Autodesk Fusion 360 part; units mm, degrees
note: some values were not read from the file. Chosen so that the rebuilt part matches the saved one: which bodies a step acts on. Set by a fixed rule: which sketch regions a step uses.
(part 3 of 6)
sketch "Sketch73" plane through (0, 0, 40) normal (0, 0, 1) x (-1, 0, 0)
  line L0 (-70.6667, -90.7407) -> (-70.6667, -70.6667)
  line L1 (-70.6667, -70.6667) -> (-90.7407, -70.6667)
  line L2 (-90.7407, -70.6667) -> (-90.7407, -67.1667)
  line L3 (-90.7407, -67.1667) -> (-109.2593, -67.1667)
  line L4 (-109.2593, -67.1667) -> (-109.2593, -70.6667)
  line L5 (-109.2593, -70.6667) -> (-129.3333, -70.6667)
  line L6 (-129.3333, -70.6667) -> (-129.3333, -88.8889)
  line L7 (-129.3333, -88.8889) -> (-137.3333, -88.8889)
  line L8 (-137.3333, -88.8889) -> (-137.3333, -70.6667)
  line L9 (-137.3333, -70.6667) -> (-157.4074, -70.6667)
  line L10 (-157.4074, -70.6667) -> (-157.4074, -67.1667)
  line L11 (-157.4074, -67.1667) -> (-175.9259, -67.1667)
  line L12 (-175.9259, -67.1667) -> (-175.9259, -70.6667)
  line L13 (-175.9259, -70.6667) -> (-196, -70.6667)
  line L14 (-196, -70.6667) -> (-196, -88.8889)
  line L15 (-196, -88.8889) -> (-200, -88.8889)
  line L16 (-200, -88.8889) -> (-200, -111.1111)
  line L17 (-200, -111.1111) -> (-196, -111.1111)
  line L18 (-196, -111.1111) -> (-196, -129.3333)
  line L19 (-196, -129.3333) -> (-177.7778, -129.3333)
  line L20 (-177.7778, -129.3333) -> (-177.7778, -137.3333)
  line L21 (-177.7778, -137.3333) -> (-196, -137.3333)
  line L22 (-196, -137.3333) -> (-196, -155.5556)
  line L23 (-196, -155.5556) -> (-200, -155.5556)
  line L24 (-200, -155.5556) -> (-200, -177.7778)
  line L25 (-200, -177.7778) -> (-196, -177.7778)
  line L26 (-196, -177.7778) -> (-196, -196)
  line L27 (-196, -196) -> (-177.7778, -196)
  line L28 (-177.7778, -196) -> (-177.7778, -200)
  line L29 (-177.7778, -200) -> (-155.5556, -200)
  line L30 (-155.5556, -200) -> (-155.5556, -196)
  line L31 (-155.5556, -196) -> (-137.3333, -196)
  line L32 (-137.3333, -196) -> (-137.3333, -177.7778)
  line L33 (-137.3333, -177.7778) -> (-129.3333, -177.7778)
  line L34 (-129.3333, -177.7778) -> (-129.3333, -196)
  line L35 (-129.3333, -196) -> (-111.1111, -196)
  line L36 (-111.1111, -196) -> (-111.1111, -200)
  line L37 (-111.1111, -200) -> (-88.8889, -200)
  line L38 (-88.8889, -200) -> (-88.8889, -196)
  line L39 (-88.8889, -196) -> (-70.6667, -196)
  line L40 (-70.6667, -196) -> (-70.6667, -177.7778)
  line L41 (-70.6667, -177.7778) -> (-62.6667, -177.7778)
  line L42 (-62.6667, -177.7778) -> (-62.6667, -196)
  line L43 (-62.6667, -196) -> (-44.4444, -196)
  line L44 (-44.4444, -196) -> (-44.4444, -200)
  line L45 (-44.4444, -200) -> (-22.2222, -200)
  line L46 (-22.2222, -200) -> (-22.2222, -196)
  line L47 (-22.2222, -196) -> (-4, -196)
  line L48 (-4, -196) -> (-4, -177.7778)
  line L49 (-4, -177.7778) -> (0, -177.7778)
  line L50 (0, -177.7778) -> (0, -155.5556)
  line L51 (0, -155.5556) -> (-4, -155.5556)
  line L52 (-4, -155.5556) -> (-4, -137.3333)
  line L53 (-4, -137.3333) -> (-24.0741, -137.3333)
  line L54 (-24.0741, -137.3333) -> (-24.0741, -133.8333)
  line L55 (-24.0741, -133.8333) -> (-42.5926, -133.8333)
  line L56 (-42.5926, -133.8333) -> (-42.5926, -137.3333)
  line L57 (-42.5926, -137.3333) -> (-62.6667, -137.3333)
  line L58 (-62.6667, -137.3333) -> (-62.6667, -155.5556)
  line L59 (-62.6667, -155.5556) -> (-70.6667, -155.5556)
  line L60 (-70.6667, -155.5556) -> (-70.6667, -137.3333)
  line L61 (-70.6667, -137.3333) -> (-88.8889, -137.3333)
  line L62 (-88.8889, -137.3333) -> (-88.8889, -129.3333)
  line L63 (-88.8889, -129.3333) -> (-70.6667, -129.3333)
  line L64 (-70.6667, -129.3333) -> (-70.6667, -109.2593)
  line L65 (-70.6667, -109.2593) -> (-67.1667, -109.2593)
  line L66 (-67.1667, -109.2593) -> (-67.1667, -90.7407)
  line L67 (-67.1667, -90.7407) -> (-70.6667, -90.7407)
  line L68 (-129.3333, -137.3333) -> (-129.3333, -155.5556)
  line L69 (-129.3333, -155.5556) -> (-137.3333, -155.5556)
  line L70 (-137.3333, -155.5556) -> (-137.3333, -137.3333)
  line L71 (-137.3333, -137.3333) -> (-155.5556, -137.3333)
  line L72 (-155.5556, -137.3333) -> (-155.5556, -129.3333)
  line L73 (-155.5556, -129.3333) -> (-137.3333, -129.3333)
  line L74 (-137.3333, -129.3333) -> (-137.3333, -111.1111)
  line L75 (-137.3333, -111.1111) -> (-129.3333, -111.1111)
  line L76 (-129.3333, -111.1111) -> (-129.3333, -129.3333)
  line L77 (-129.3333, -129.3333) -> (-111.1111, -129.3333)
  line L78 (-111.1111, -129.3333) -> (-111.1111, -137.3333)
  line L79 (-111.1111, -137.3333) -> (-129.3333, -137.3333)
  line L80 (-88.8889, -137.3333) -> (-90.7407, -137.3333)
  line L81 (-90.7407, -137.3333) -> (-90.7407, -129.3333)
  line L82 (-90.7407, -129.3333) -> (-88.8889, -129.3333)
  line L83 (-88.8889, -129.3333) -> (-88.8889, -137.3333)
  line L84 (-111.1111, -137.3333) -> (-109.2593, -137.3333)
  line L85 (-109.2593, -137.3333) -> (-109.2593, -129.3333)
  line L86 (-109.2593, -129.3333) -> (-111.1111, -129.3333)
  line L87 (-111.1111, -129.3333) -> (-111.1111, -137.3333)
  line L88 (-88.8889, -133.8333) -> (-111.1111, -133.8333)
  line L89 (-111.1111, -133.8333) -> (-111.1111, -132.8333)
  line L90 (-111.1111, -132.8333) -> (-88.8889, -132.8333)
  line L91 (-88.8889, -132.8333) -> (-88.8889, -133.8333)
  line L92 (-129.3333, -111.1111) -> (-137.3333, -111.1111)
  line L93 (-137.3333, -111.1111) -> (-137.3333, -109.2593)
  line L94 (-137.3333, -109.2593) -> (-129.3333, -109.2593)
  line L95 (-129.3333, -109.2593) -> (-129.3333, -111.1111)
  line L96 (-129.3333, -88.8889) -> (-137.3333, -88.8889)
  line L97 (-137.3333, -88.8889) -> (-137.3333, -90.7407)
  line L98 (-137.3333, -90.7407) -> (-129.3333, -90.7407)
  line L99 (-129.3333, -90.7407) -> (-129.3333, -88.8889)
  line L100 (-132.8333, -111.1111) -> (-133.8333, -111.1111)
  line L101 (-133.8333, -111.1111) -> (-133.8333, -88.8889)
  line L102 (-133.8333, -88.8889) -> (-132.8333, -88.8889)
  line L103 (-132.8333, -88.8889) -> (-132.8333, -111.1111)
  dimension "d406" = 1.8519
  dimension "d407" = 1.8519
  dimension "d408" = 8
  dimension "d409" = 8
  dimension "d410" = 22.2222
  dimension "d411" = 1
  dimension "d412" = 3.5
  dimension "d413" = 8
  dimension "d414" = 1.8519
  dimension "d415" = 1.8519
  dimension "d416" = 8
  dimension "d421" = 1
  dimension "d422" = 3.5
  dimension "d423" = 22.2222
  constraint horizontal L80
  constraint vertical L81
  constraint horizontal L82
  constraint vertical L83
  constraint coincident L61.end L62.start
  constraint horizontal L84
  constraint vertical L85
  constraint horizontal L86
  constraint vertical L87
  constraint coincident L78.end L79.start
  constraint horizontal L88
  constraint vertical L89
  constraint horizontal L90
  constraint vertical L91
  constraint coincident L83 L88.start
  constraint horizontal L92
  constraint vertical L93
  constraint horizontal L94
  constraint vertical L95
  constraint coincident L75.end L76.start
  constraint horizontal L96
  constraint vertical L97
  constraint horizontal L98
  constraint vertical L99
  constraint coincident L6.end L7.start
  constraint horizontal L100
  constraint vertical L101
  constraint horizontal L102
  constraint vertical L103
  constraint coincident L75 L100.start
  measures "d406" distance of L81.end L62.end
  measures "d407" distance of L85.end L77.end
  measures "d408" distance of L78.end L77.end
  measures "d409" distance of L61.end L62.end
  measures "d410" distance of L89.end L90.end
  measures "d411" distance of L88.end L89.end
  measures "d412" distance of L78.end L88.end
  measures "d413" distance of L6.end L7.end
  measures "d414" distance of L7.end L97.end
  measures "d415" distance of L74.end L93.end
  measures "d416" distance of L93.end L94.end
  measures "d421" distance of L101.end L102.end
  measures "d422" distance of L6.end L103
  measures "d423" distance of L100.end L101.end
extrude "Extrude42" cut sketch "Sketch73" against normal blind 4 contours L62 L81 L82 L83 L90 | L62 L81 L83 L88 L90 L91 | L7 L96 L98 L99 L103 | L62 L80 L81 L83 L88 | L81 L85 L88 L90 | L7 L96 L98 L101 L102 L103 | L78 L85 L86 L87 L90 | L78 L85 L87 L88 L89 L90 | L7 L96 L97 L98 L101 | L94 L98 L101 L103 | L78 L84 L85 L87 L88 | L75 L92 L94 L100 L101 L103 | L75 L92 L94 L95 L103 | L75 L92 L93 L94 L101 bodies 17 makes body 18 at (163.679, 103.0864, 40)
sketch "Sketch74" plane through (0, 0, 40) normal (0, 0, 1) x (-1, 0, 0)
  line L0 (-109.2593, -137.3333) -> (-129.3333, -137.3333)
  line L1 (-129.3333, -137.3333) -> (-129.3333, -155.5556)
  line L2 (-129.3333, -155.5556) -> (-137.3333, -155.5556)
  line L3 (-137.3333, -155.5556) -> (-137.3333, -137.3333)
  line L4 (-137.3333, -137.3333) -> (-155.5556, -137.3333)
  line L5 (-155.5556, -137.3333) -> (-155.5556, -129.3333)
  line L6 (-155.5556, -129.3333) -> (-137.3333, -129.3333)
  line L7 (-137.3333, -129.3333) -> (-137.3333, -109.2593)
  line L8 (-137.3333, -109.2593) -> (-133.8333, -109.2593)
  line L9 (-133.8333, -109.2593) -> (-133.8333, -90.7407)
  line L10 (-133.8333, -90.7407) -> (-137.3333, -90.7407)
  line L11 (-137.3333, -90.7407) -> (-137.3333, -70.6667)
  line L12 (-137.3333, -70.6667) -> (-157.4074, -70.6667)
  line L13 (-157.4074, -70.6667) -> (-157.4074, -67.1667)
  line L14 (-157.4074, -67.1667) -> (-175.9259, -67.1667)
  line L15 (-175.9259, -67.1667) -> (-175.9259, -70.6667)
  line L16 (-175.9259, -70.6667) -> (-196, -70.6667)
  line L17 (-196, -70.6667) -> (-196, -88.8889)
  line L18 (-196, -88.8889) -> (-200, -88.8889)
  line L19 (-200, -88.8889) -> (-200, -111.1111)
  line L20 (-200, -111.1111) -> (-196, -111.1111)
  line L21 (-196, -111.1111) -> (-196, -129.3333)
  line L22 (-196, -129.3333) -> (-177.7778, -129.3333)
  line L23 (-177.7778, -129.3333) -> (-177.7778, -137.3333)
  line L24 (-177.7778, -137.3333) -> (-196, -137.3333)
  line L25 (-196, -137.3333) -> (-196, -155.5556)
  line L26 (-196, -155.5556) -> (-200, -155.5556)
  line L27 (-200, -155.5556) -> (-200, -177.7778)
  line L28 (-200, -177.7778) -> (-196, -177.7778)
  line L29 (-196, -177.7778) -> (-196, -196)
  line L30 (-196, -196) -> (-177.7778, -196)
  line L31 (-177.7778, -196) -> (-177.7778, -200)
  line L32 (-177.7778, -200) -> (-155.5556, -200)
  line L33 (-155.5556, -200) -> (-155.5556, -196)
  line L34 (-155.5556, -196) -> (-137.3333, -196)
  line L35 (-137.3333, -196) -> (-137.3333, -177.7778)
  line L36 (-137.3333, -177.7778) -> (-129.3333, -177.7778)
  line L37 (-129.3333, -177.7778) -> (-129.3333, -196)
  line L38 (-129.3333, -196) -> (-111.1111, -196)
  line L39 (-111.1111, -196) -> (-111.1111, -200)
  line L40 (-111.1111, -200) -> (-88.8889, -200)
  line L41 (-88.8889, -200) -> (-88.8889, -196)
  line L42 (-88.8889, -196) -> (-70.6667, -196)
  line L43 (-70.6667, -196) -> (-70.6667, -177.7778)
  line L44 (-70.6667, -177.7778) -> (-62.6667, -177.7778)
  line L45 (-62.6667, -177.7778) -> (-62.6667, -196)
  line L46 (-62.6667, -196) -> (-44.4444, -196)
  line L47 (-44.4444, -196) -> (-44.4444, -200)
  line L48 (-44.4444, -200) -> (-22.2222, -200)
  line L49 (-22.2222, -200) -> (-22.2222, -196)
  line L50 (-22.2222, -196) -> (-4, -196)
  line L51 (-4, -196) -> (-4, -177.7778)
  line L52 (-4, -177.7778) -> (0, -177.7778)
  line L53 (0, -177.7778) -> (0, -155.5556)
  line L54 (0, -155.5556) -> (-4, -155.5556)
  line L55 (-4, -155.5556) -> (-4, -137.3333)
  line L56 (-4, -137.3333) -> (-24.0741, -137.3333)
  line L57 (-24.0741, -137.3333) -> (-24.0741, -133.8333)
  line L58 (-24.0741, -133.8333) -> (-42.5926, -133.8333)
  line L59 (-42.5926, -133.8333) -> (-42.5926, -137.3333)
  line L60 (-42.5926, -137.3333) -> (-62.6667, -137.3333)
  line L61 (-62.6667, -137.3333) -> (-62.6667, -155.5556)
  line L62 (-62.6667, -155.5556) -> (-70.6667, -155.5556)
  line L63 (-70.6667, -155.5556) -> (-70.6667, -137.3333)
  line L64 (-70.6667, -137.3333) -> (-90.7407, -137.3333)
  line L65 (-90.7407, -137.3333) -> (-90.7407, -133.8333)
  line L66 (-90.7407, -133.8333) -> (-109.2593, -133.8333)
  line L67 (-109.2593, -133.8333) -> (-109.2593, -137.3333)
  line L68 (-155.5556, -137.3333) -> (-157.4074, -137.3333)
  line L69 (-157.4074, -137.3333) -> (-157.4074, -129.3333)
  line L70 (-157.4074, -129.3333) -> (-155.5556, -129.3333)
  line L71 (-155.5556, -129.3333) -> (-155.5556, -137.3333)
  line L72 (-177.7778, -137.3333) -> (-175.9259, -137.3333)
  line L73 (-175.9259, -137.3333) -> (-175.9259, -129.3333)
  line L74 (-175.9259, -129.3333) -> (-177.7778, -129.3333)
  line L75 (-177.7778, -129.3333) -> (-177.7778, -137.3333)
  line L76 (-155.5556, -133.8333) -> (-177.7778, -133.8333)
  line L77 (-177.7778, -133.8333) -> (-177.7778, -132.8333)
  line L78 (-177.7778, -132.8333) -> (-155.5556, -132.8333)
  line L79 (-155.5556, -132.8333) -> (-155.5556, -133.8333)
  line L80 (-196, -111.1111) -> (-199.5, -111.1111)
  line L81 (-199.5, -111.1111) -> (-199.5, -109.2593)
  line L82 (-199.5, -109.2593) -> (-196, -109.2593)
  line L83 (-196, -109.2593) -> (-196, -111.1111)
  line L84 (-200, -111.1111) -> (-199.5, -111.1111)
  line L85 (-199.5, -111.1111) -> (-199.5, -88.8889)
  line L86 (-199.5, -88.8889) -> (-200, -88.8889)
  line L87 (-200, -88.8889) -> (-200, -111.1111)
  line L88 (-196, -88.8889) -> (-199.5, -88.8889)
  line L89 (-199.5, -88.8889) -> (-199.5, -90.7407)
  line L90 (-199.5, -90.7407) -> (-196, -90.7407)
  line L91 (-196, -90.7407) -> (-196, -88.8889)
  dimension "d426" = 1.8519
  dimension "d427" = 3.5
  dimension "d428" = 0.5
  dimension "d429" = 22.2222
  dimension "d430" = 1.8519
  dimension "d431" = 3.5
  dimension "d432" = 1.8519
  dimension "d433" = 1.8519
  dimension "d434" = 8
  dimension "d435" = 8
  dimension "d436" = 3.5
  dimension "d437" = 1
  dimension "d438" = 22.2222
  constraint horizontal L68
  constraint vertical L69
  constraint horizontal L70
  constraint vertical L71
  constraint coincident L4.end L5.start
  constraint horizontal L72
  constraint vertical L73
  constraint horizontal L74
  constraint vertical L75
  constraint coincident L23.end L24.start
  constraint horizontal L76
  constraint vertical L77
  constraint horizontal L78
  constraint vertical L79
  constraint coincident L5 L76.start
  constraint horizontal L80
  constraint vertical L81
  constraint horizontal L82
  constraint vertical L83
  constraint coincident L20.end L21.start
  constraint horizontal L84
  constraint vertical L85
  constraint horizontal L86
  constraint vertical L87
  constraint coincident L19.end L20.start
  constraint horizontal L88
  constraint vertical L89
  constraint horizontal L90
  constraint vertical L91
  constraint coincident L17.end L18.start
  measures "d426" distance of L80.end L81.end
  measures "d427" distance of L20.end L80.end
  measures "d428" distance of L19.end L80.end
  measures "d429" distance of L19.end L18.end
  measures "d430" distance of L85.end L89.end
  measures "d431" distance of L17.end L85.end
  measures "d432" distance of L69.end L5.end
  measures "d433" distance of L73.end L22.end
  measures "d434" distance of L23.end L22.end
  measures "d435" distance of L4.end L5.end
  measures "d436" distance of L5.end L78.end
  measures "d437" distance of L76.start L78.end
  measures "d438" distance of L77.end L78.end
extrude "Extrude43" cut sketch "Sketch74" against normal blind 4 contours L5 L68 L69 L71 L76 | L5 L69 L71 L76 L78 L79 | L5 L69 L70 L71 L78 | L69 L73 L76 L78 | L23 L73 L75 L76 L77 L78 | L23 L72 L73 L75 L76 | L23 L73 L74 L75 L78 | L20 L80 L81 L82 L83 L85 | L18 L19 L20 L81 L84 L85 L86 L87 L89 | L18 L85 L88 L89 L90 L91 bodies 18 makes body 19 at (163.5802, 176.4444, 40)
sketch "Sketch75" plane through (0, 0, 40) normal (0, 0, 1) x (-1, 0, 0)
  line L0 (-137.3333, -137.3333) -> (-157.4074, -137.3333)
  line L1 (-157.4074, -137.3333) -> (-157.4074, -133.8333)
  line L2 (-157.4074, -133.8333) -> (-175.9259, -133.8333)
  line L3 (-175.9259, -133.8333) -> (-175.9259, -137.3333)
  line L4 (-175.9259, -137.3333) -> (-196, -137.3333)
  line L5 (-196, -137.3333) -> (-196, -155.5556)
  line L6 (-196, -155.5556) -> (-200, -155.5556)
  line L7 (-200, -155.5556) -> (-200, -177.7778)
  line L8 (-200, -177.7778) -> (-196, -177.7778)
  line L9 (-196, -177.7778) -> (-196, -196)
  line L10 (-196, -196) -> (-177.7778, -196)
  line L11 (-177.7778, -196) -> (-177.7778, -200)
  line L12 (-177.7778, -200) -> (-155.5556, -200)
  line L13 (-155.5556, -200) -> (-155.5556, -196)
  line L14 (-155.5556, -196) -> (-137.3333, -196)
  line L15 (-137.3333, -196) -> (-137.3333, -177.7778)
  line L16 (-137.3333, -177.7778) -> (-129.3333, -177.7778)
  line L17 (-129.3333, -177.7778) -> (-129.3333, -196)
  line L18 (-129.3333, -196) -> (-111.1111, -196)
  line L19 (-111.1111, -196) -> (-111.1111, -200)
  line L20 (-111.1111, -200) -> (-88.8889, -200)
  line L21 (-88.8889, -200) -> (-88.8889, -196)
  line L22 (-88.8889, -196) -> (-70.6667, -196)
  line L23 (-70.6667, -196) -> (-70.6667, -177.7778)
  line L24 (-70.6667, -177.7778) -> (-62.6667, -177.7778)
  line L25 (-62.6667, -177.7778) -> (-62.6667, -196)
  line L26 (-62.6667, -196) -> (-44.4444, -196)
  line L27 (-44.4444, -196) -> (-44.4444, -200)
  line L28 (-44.4444, -200) -> (-22.2222, -200)
  line L29 (-22.2222, -200) -> (-22.2222, -196)
  line L30 (-22.2222, -196) -> (-4, -196)
  line L31 (-4, -196) -> (-4, -177.7778)
  line L32 (-4, -177.7778) -> (0, -177.7778)
  line L33 (0, -177.7778) -> (0, -155.5556)
  line L34 (0, -155.5556) -> (-4, -155.5556)
  line L35 (-4, -155.5556) -> (-4, -137.3333)
  line L36 (-4, -137.3333) -> (-24.0741, -137.3333)
  line L37 (-24.0741, -137.3333) -> (-24.0741, -133.8333)
  line L38 (-24.0741, -133.8333) -> (-42.5926, -133.8333)
  line L39 (-42.5926, -133.8333) -> (-42.5926, -137.3333)
  line L40 (-42.5926, -137.3333) -> (-62.6667, -137.3333)
  line L41 (-62.6667, -137.3333) -> (-62.6667, -155.5556)
  line L42 (-62.6667, -155.5556) -> (-70.6667, -155.5556)
  line L43 (-70.6667, -155.5556) -> (-70.6667, -137.3333)
  line L44 (-70.6667, -137.3333) -> (-90.7407, -137.3333)
  line L45 (-90.7407, -137.3333) -> (-90.7407, -133.8333)
  line L46 (-90.7407, -133.8333) -> (-109.2593, -133.8333)
  line L47 (-109.2593, -133.8333) -> (-109.2593, -137.3333)
  line L48 (-109.2593, -137.3333) -> (-129.3333, -137.3333)
  line L49 (-129.3333, -137.3333) -> (-129.3333, -155.5556)
  line L50 (-129.3333, -155.5556) -> (-137.3333, -155.5556)
  line L51 (-137.3333, -155.5556) -> (-137.3333, -137.3333)
  line L52 (-4, -177.7778) -> (-0.5, -177.7778)
  line L53 (-0.5, -177.7778) -> (-0.5, -175.9259)
  line L54 (-0.5, -175.9259) -> (-4, -175.9259)
  line L55 (-4, -175.9259) -> (-4, -177.7778)
  line L56 (-4, -155.5556) -> (-0.5, -155.5556)
  line L57 (-0.5, -155.5556) -> (-0.5, -157.4074)
  line L58 (-0.5, -157.4074) -> (-4, -157.4074)
  line L59 (-4, -157.4074) -> (-4, -155.5556)
  line L60 (0, -177.7778) -> (-0.5, -177.7778)
  line L61 (-0.5, -177.7778) -> (-0.5, -155.5556)
  line L62 (-0.5, -155.5556) -> (0, -155.5556)
  line L63 (0, -155.5556) -> (0, -177.7778)
  line L64 (-62.6667, -177.7778) -> (-70.6667, -177.7778)
  line L65 (-70.6667, -177.7778) -> (-70.6667, -175.9259)
  line L66 (-70.6667, -175.9259) -> (-62.6667, -175.9259)
  line L67 (-62.6667, -175.9259) -> (-62.6667, -177.7778)
  line L68 (-62.6667, -155.5556) -> (-70.6667, -155.5556)
  line L69 (-70.6667, -155.5556) -> (-70.6667, -157.4074)
  line L70 (-70.6667, -157.4074) -> (-62.6667, -157.4074)
  line L71 (-62.6667, -157.4074) -> (-62.6667, -155.5556)
  line L72 (-66.1667, -177.7778) -> (-67.1667, -177.7778)
  line L73 (-67.1667, -177.7778) -> (-67.1667, -155.5556)
  line L74 (-67.1667, -155.5556) -> (-66.1667, -155.5556)
  line L75 (-66.1667, -155.5556) -> (-66.1667, -177.7778)
  line L76 (-22.2222, -196) -> (-24.0741, -196)
  line L77 (-24.0741, -196) -> (-24.0741, -199.5)
  line L78 (-24.0741, -199.5) -> (-22.2222, -199.5)
  line L79 (-22.2222, -199.5) -> (-22.2222, -196)
  line L80 (-44.4444, -196) -> (-42.5926, -196)
  line L81 (-42.5926, -196) -> (-42.5926, -199.5)
  line L82 (-42.5926, -199.5) -> (-44.4444, -199.5)
  line L83 (-44.4444, -199.5) -> (-44.4444, -196)
  line L84 (-22.2222, -200) -> (-44.4444, -200)
  line L85 (-44.4444, -200) -> (-44.4444, -199.5)
  line L86 (-44.4444, -199.5) -> (-22.2222, -199.5)
  line L87 (-22.2222, -199.5) -> (-22.2222, -200)
  dimension "d441" = 1.8519
  dimension "d442" = 1.8519
  dimension "d443" = 3.5
  dimension "d444" = 3.5
  dimension "d445" = 0.5
  dimension "d446" = 22.2222
  dimension "d447" = 1.8519
  dimension "d448" = 1.8519
  dimension "d449" = 1
  dimension "d450" = 22.2222
  dimension "d451" = 3.5
  dimension "d452" = 8
  dimension "d453" = 8
  dimension "d454" = 1.8519
  dimension "d455" = 1.8519
  dimension "d456" = 3.5
  dimension "d457" = 3.5
  dimension "d458" = 22.2222
  dimension "d459" = 0.5
  dimension "d460" = 22.2222
  constraint horizontal L52
  constraint vertical L53
  constraint horizontal L54
  constraint vertical L55
  constraint coincident L31.end L32.start
  constraint horizontal L56
  constraint vertical L57
  constraint horizontal L58
  constraint vertical L59
  constraint coincident L34.end L35.start
  constraint horizontal L60
  constraint vertical L61
  constraint horizontal L62
  constraint vertical L63
  constraint coincident L32.end L33.start
  constraint horizontal L64
  constraint vertical L65
  constraint horizontal L66
  constraint vertical L67
  constraint coincident L24.end L25.start
  constraint horizontal L68
  constraint vertical L69
  constraint horizontal L70
  constraint vertical L71
  constraint coincident L41.end L42.start
  constraint horizontal L72
  constraint vertical L73
  constraint horizontal L74
  constraint vertical L75
  constraint coincident L64 L72.start
  constraint horizontal L76
  constraint vertical L77
  constraint horizontal L78
  constraint vertical L79
  constraint coincident L29.end L30.start
  constraint horizontal L80
  constraint vertical L81
  constraint horizontal L82
  constraint vertical L83
  constraint coincident L26.end L27.start
  constraint horizontal L84
  constraint vertical L85
  constraint horizontal L86
  constraint vertical L87
  constraint coincident L28.end L29.start
  measures "d441" distance of L31.end L54.end
  measures "d442" distance of L34.end L58.end
  measures "d443" distance of L34.end L56.end
  measures "d444" distance of L31.end L52.end
  measures "d445" distance of L56.end L33.end
  measures "d446" distance of L32.end L33.end
  measures "d447" distance of L23.end L65.end
  measures "d448" distance of L42.end L69.end
  measures "d449" distance of L73.end L74.end
  measures "d450" distance of L72.end L73.end
  measures "d451" distance of L24.end L72.start
  measures "d452" distance of L65.end L66.end
  measures "d453" distance of L69.end L70.end
  measures "d454" distance of L26.end L80.end
  measures "d455" distance of L29.end L76.end
  measures "d456" distance of L29.end L78.end
  measures "d457" distance of L26.end L82.end
  measures "d458" distance of L82.end L78.end
  measures "d459" distance of L28.end L78.end
  measures "d460" distance of L28.end L27.end
extrude "Extrude44" cut sketch "Sketch75" against normal blind 4 contours L42 L68 L69 L70 L73 | L42 L68 L70 L73 L74 L75 | L42 L68 L70 L71 L75 | L66 L70 L73 L75 | L24 L64 L65 L66 L73 | L24 L64 L66 L72 L73 L75 | L24 L64 L66 L67 L75 | L27 L80 L81 L82 L83 L86 | L27 L28 L29 L78 L82 L84 L85 L86 L87 | L34 L56 L57 L58 L59 L61 | L32 L33 L34 L53 L57 L60 L61 L62 L63 | L29 L76 L77 L78 L79 L86 | L32 L52 L53 L54 L55 L61 bodies 19 makes body 20 at (97.0123, 169.7531, 40)
sketch "Sketch76" plane through (0, 0, 40) normal (0, 0, 1) x (-1, 0, 0)
  line L0 (-70.6667, -196) -> (-70.6667, -175.9259)
  line L1 (-70.6667, -175.9259) -> (-67.1667, -175.9259)
  line L2 (-67.1667, -175.9259) -> (-67.1667, -157.4074)
  line L3 (-67.1667, -157.4074) -> (-70.6667, -157.4074)
  line L4 (-70.6667, -157.4074) -> (-70.6667, -137.3333)
  line L5 (-70.6667, -137.3333) -> (-90.7407, -137.3333)
  line L6 (-90.7407, -137.3333) -> (-90.7407, -133.8333)
  line L7 (-90.7407, -133.8333) -> (-109.2593, -133.8333)
  line L8 (-109.2593, -133.8333) -> (-109.2593, -137.3333)
  line L9 (-109.2593, -137.3333) -> (-129.3333, -137.3333)
  line L10 (-129.3333, -137.3333) -> (-129.3333, -155.5556)
  line L11 (-129.3333, -155.5556) -> (-137.3333, -155.5556)
  line L12 (-137.3333, -155.5556) -> (-137.3333, -137.3333)
  line L13 (-137.3333, -137.3333) -> (-157.4074, -137.3333)
  line L14 (-157.4074, -137.3333) -> (-157.4074, -133.8333)
  line L15 (-157.4074, -133.8333) -> (-175.9259, -133.8333)
  line L16 (-175.9259, -133.8333) -> (-175.9259, -137.3333)
  line L17 (-175.9259, -137.3333) -> (-196, -137.3333)
  line L18 (-196, -137.3333) -> (-196, -155.5556)
  line L19 (-196, -155.5556) -> (-200, -155.5556)
  line L20 (-200, -155.5556) -> (-200, -177.7778)
  line L21 (-200, -177.7778) -> (-196, -177.7778)
  line L22 (-196, -177.7778) -> (-196, -196)
  line L23 (-196, -196) -> (-177.7778, -196)
  line L24 (-177.7778, -196) -> (-177.7778, -200)
  line L25 (-177.7778, -200) -> (-155.5556, -200)
  line L26 (-155.5556, -200) -> (-155.5556, -196)
  line L27 (-155.5556, -196) -> (-137.3333, -196)
  line L28 (-137.3333, -196) -> (-137.3333, -177.7778)
  line L29 (-137.3333, -177.7778) -> (-129.3333, -177.7778)
  line L30 (-129.3333, -177.7778) -> (-129.3333, -196)
  line L31 (-129.3333, -196) -> (-111.1111, -196)
  line L32 (-111.1111, -196) -> (-111.1111, -200)
  line L33 (-111.1111, -200) -> (-88.8889, -200)
  line L34 (-88.8889, -200) -> (-88.8889, -196)
  line L35 (-88.8889, -196) -> (-70.6667, -196)
  line L36 (-88.8889, -196) -> (-90.7407, -196)
  line L37 (-90.7407, -196) -> (-90.7407, -199.5)
  line L38 (-90.7407, -199.5) -> (-88.8889, -199.5)
  line L39 (-88.8889, -199.5) -> (-88.8889, -196)
  line L40 (-111.1111, -196) -> (-109.2593, -196)
  line L41 (-109.2593, -196) -> (-109.2593, -199.5)
  line L42 (-109.2593, -199.5) -> (-111.1111, -199.5)
  line L43 (-111.1111, -199.5) -> (-111.1111, -196)
  line L44 (-88.8889, -200) -> (-111.1111, -200)
  line L45 (-111.1111, -200) -> (-111.1111, -199.5)
  line L46 (-111.1111, -199.5) -> (-88.8889, -199.5)
  line L47 (-88.8889, -199.5) -> (-88.8889, -200)
  line L48 (-129.3333, -177.7778) -> (-137.3333, -177.7778)
  line L49 (-137.3333, -177.7778) -> (-137.3333, -175.9259)
  line L50 (-137.3333, -175.9259) -> (-129.3333, -175.9259)
  line L51 (-129.3333, -175.9259) -> (-129.3333, -177.7778)
  line L52 (-132.8333, -177.7778) -> (-133.8333, -177.7778)
  line L53 (-133.8333, -177.7778) -> (-133.8333, -155.5556)
  line L54 (-133.8333, -155.5556) -> (-132.8333, -155.5556)
  line L55 (-132.8333, -155.5556) -> (-132.8333, -177.7778)
  line L56 (-129.3333, -155.5556) -> (-137.3333, -155.5556)
  line L57 (-137.3333, -155.5556) -> (-137.3333, -157.4074)
  line L58 (-137.3333, -157.4074) -> (-129.3333, -157.4074)
  line L59 (-129.3333, -157.4074) -> (-129.3333, -155.5556)
  dimension "d463" = 1.8519
  dimension "d464" = 1.8519
  dimension "d465" = 3.5
  dimension "d466" = 22.2222
  dimension "d467" = 3.5
  dimension "d468" = 0.5
  dimension "d469" = 1
  dimension "d470" = 8
  dimension "d471" = 1.8519
  dimension "d472" = 22.2222
  dimension "d473" = 3.5
  dimension "d474" = 1.8519
  dimension "d475" = 8
  dimension "d476" = 3.5
  constraint horizontal L36
  constraint vertical L37
  constraint horizontal L38
  constraint vertical L39
  constraint coincident L34.end L35.start
  constraint horizontal L40
  constraint vertical L41
  constraint horizontal L42
  constraint vertical L43
  constraint coincident L31.end L32.start
  constraint horizontal L44
  constraint vertical L45
  constraint horizontal L46
  constraint vertical L47
  constraint coincident L33.end L34.start
  constraint horizontal L48
  constraint vertical L49
  constraint horizontal L50
  constraint vertical L51
  constraint coincident L29.end L30.start
  constraint horizontal L52
  constraint vertical L53
  constraint horizontal L54
  constraint vertical L55
  constraint coincident L48 L52.start
  constraint horizontal L56
  constraint vertical L57
  constraint horizontal L58
  constraint vertical L59
  constraint coincident L10.end L11.start
  measures "d463" distance of L34.end L36.end
  measures "d464" distance of L31.end L40.end
  measures "d465" distance of L31.end L42.end
  measures "d466" distance of L42.end L38.end
  measures "d467" distance of L34.end L38.end
  measures "d468" distance of L33.end L38.end
  measures "d469" distance of L53.end L54.end
  measures "d470" distance of L10.end L11.end
  measures "d471" distance of L11.end L57.end
  measures "d472" distance of L52.end L53.end
  measures "d473" distance of L11.end L53.end
  measures "d474" distance of L29.end L50.end
  measures "d475" distance of L49.end L50.end
  measures "d476" distance of L49.end L53
extrude "Extrude45" cut sketch "Sketch76" against normal blind 4 contours L34 L36 L37 L38 L39 L46 | L32 L33 L34 L38 L42 L44 L45 L46 L47 | L32 L40 L41 L42 L43 L46 | L29 L48 L50 L51 L55 | L29 L48 L50 L52 L53 L55 | L29 L48 L49 L50 L53 | L50 L53 L55 L58 | L11 L55 L56 L58 L59 | L11 L53 L54 L55 L56 L58 | L11 L53 L56 L57 L58 bodies 20 makes body 21 at (163.679, 169.7531, 40)
sketch "Sketch77" plane through (0, 0, 40) normal (0, 0, 1) x (-1, 0, 0)
  line L0 (-137.3333, -157.4074) -> (-137.3333, -137.3333)
  line L1 (-137.3333, -137.3333) -> (-157.4074, -137.3333)
  line L2 (-157.4074, -137.3333) -> (-157.4074, -133.8333)
  line L3 (-157.4074, -133.8333) -> (-175.9259, -133.8333)
  line L4 (-175.9259, -133.8333) -> (-175.9259, -137.3333)
  line L5 (-175.9259, -137.3333) -> (-196, -137.3333)
  line L6 (-196, -137.3333) -> (-196, -155.5556)
  line L7 (-196, -155.5556) -> (-200, -155.5556)
  line L8 (-200, -155.5556) -> (-200, -177.7778)
  line L9 (-200, -177.7778) -> (-196, -177.7778)
  line L10 (-196, -177.7778) -> (-196, -196)
  line L11 (-196, -196) -> (-177.7778, -196)
  line L12 (-177.7778, -196) -> (-177.7778, -200)
  line L13 (-177.7778, -200) -> (-155.5556, -200)
  line L14 (-155.5556, -200) -> (-155.5556, -196)
  line L15 (-155.5556, -196) -> (-137.3333, -196)
  line L16 (-137.3333, -196) -> (-137.3333, -175.9259)
  line L17 (-137.3333, -175.9259) -> (-133.8333, -175.9259)
  line L18 (-133.8333, -175.9259) -> (-133.8333, -157.4074)
  line L19 (-133.8333, -157.4074) -> (-137.3333, -157.4074)
  line L20 (-155.5556, -196) -> (-157.4074, -196)
  line L21 (-157.4074, -196) -> (-157.4074, -199.5)
  line L22 (-157.4074, -199.5) -> (-155.5556, -199.5)
  line L23 (-155.5556, -199.5) -> (-155.5556, -196)
  line L24 (-177.7778, -196) -> (-175.9259, -196)
  line L25 (-175.9259, -196) -> (-175.9259, -199.5)
  line L26 (-175.9259, -199.5) -> (-177.7778, -199.5)
  line L27 (-177.7778, -199.5) -> (-177.7778, -196)
  line L28 (-155.5556, -200) -> (-177.7778, -200)
  line L29 (-177.7778, -200) -> (-177.7778, -199.5)
  line L30 (-177.7778, -199.5) -> (-155.5556, -199.5)
  line L31 (-155.5556, -199.5) -> (-155.5556, -200)
  line L32 (-196, -177.7778) -> (-199.5, -177.7778)
  line L33 (-199.5, -177.7778) -> (-199.5, -175.9259)
  line L34 (-199.5, -175.9259) -> (-196, -175.9259)
  line L35 (-196, -175.9259) -> (-196, -177.7778)
  line L36 (-196, -155.5556) -> (-199.5, -155.5556)
  line L37 (-199.5, -155.5556) -> (-199.5, -157.4074)
  line L38 (-199.5, -157.4074) -> (-196, -157.4074)
  line L39 (-196, -157.4074) -> (-196, -155.5556)
  line L40 (-200, -177.7778) -> (-199.5, -177.7778)
  line L41 (-199.5, -177.7778) -> (-199.5, -155.5556)
  line L42 (-199.5, -155.5556) -> (-200, -155.5556)
  line L43 (-200, -155.5556) -> (-200, -177.7778)
  dimension "d479" = 3.5
  dimension "d480" = 22.2222
  dimension "d481" = 0.5
  dimension "d482" = 1.8519
  dimension "d483" = 1.8519
  dimension "d484" = 3.5
  dimension "d485" = 3.5
  dimension "d486" = 1.8519
  dimension "d487" = 1.8519
  dimension "d488" = 3.5
  dimension "d489" = 0.5
  dimension "d490" = 22.2222
  constraint horizontal L20
  constraint vertical L21
  constraint horizontal L22
  constraint vertical L23
  constraint coincident L14.end L15.start
  constraint horizontal L24
  constraint vertical L25
  constraint horizontal L26
  constraint vertical L27
  constraint coincident L11.end L12.start
  constraint horizontal L28
  constraint vertical L29
  constraint horizontal L30
  constraint vertical L31
  constraint coincident L13.end L14.start
  constraint horizontal L32
  constraint vertical L33
  constraint horizontal L34
  constraint vertical L35
  constraint coincident L9.end L10.start
  constraint horizontal L36
  constraint vertical L37
  constraint horizontal L38
  constraint vertical L39
  constraint coincident L6.end L7.start
  constraint horizontal L40
  constraint vertical L41
  constraint horizontal L42
  constraint vertical L43
  constraint coincident L8.end L9.start
  measures "d479" distance of L11.end L26.end
  measures "d480" distance of L26.end L22.end
  measures "d481" distance of L12.end L26.end
  measures "d482" distance of L11.end L24.end
  measures "d483" distance of L14.end L20.end
  measures "d484" distance of L20.end L21.end
  measures "d485" distance of L33.end L34.end
  measures "d486" distance of L9.end L34.end
  measures "d487" distance of L6.end L38.end
  measures "d488" distance of L6.end L36.end
  measures "d489" distance of L36.end L7.end
  measures "d490" distance of L8.end L7.end
extrude "Extrude46" cut sketch "Sketch77" against normal blind 4 contours L14 L20 L21 L22 L23 L30 | L12 L13 L14 L22 L26 L28 L29 L30 L31 | L7 L36 L37 L38 L39 L41 | L7 L8 L9 L33 L37 L40 L41 L42 L43 | L12 L24 L25 L26 L27 L30 | L9 L32 L33 L34 L35 L41 bodies 21
sketch "Sketch78" plane through (0, 0, 40) normal (0, 0, 1) x (-1, 0, 0)
  line L0 (-4, -24.0741) -> (-4, -4)
  line L1 (-4, -4) -> (-24.0741, -4)
  line L2 (-24.0741, -4) -> (-24.0741, -0.5)
  line L3 (-24.0741, -0.5) -> (-42.5926, -0.5)
  line L4 (-42.5926, -0.5) -> (-42.5926, -4)
  line L5 (-42.5926, -4) -> (-62.6667, -4)
  line L6 (-62.6667, -4) -> (-62.6667, -24.0741)
  line L7 (-62.6667, -24.0741) -> (-66.1667, -24.0741)
  line L8 (-66.1667, -24.0741) -> (-66.1667, -42.5926)
  line L9 (-66.1667, -42.5926) -> (-62.6667, -42.5926)
  line L10 (-62.6667, -42.5926) -> (-62.6667, -62.6667)
  line L11 (-62.6667, -62.6667) -> (-42.5926, -62.6667)
  line L12 (-42.5926, -62.6667) -> (-42.5926, -66.1667)
  line L13 (-42.5926, -66.1667) -> (-24.0741, -66.1667)
  line L14 (-24.0741, -66.1667) -> (-24.0741, -62.6667)
  line L15 (-24.0741, -62.6667) -> (-4, -62.6667)
  line L16 (-4, -62.6667) -> (-4, -42.5926)
  line L17 (-4, -42.5926) -> (-0.5, -42.5926)
  line L18 (-0.5, -42.5926) -> (-0.5, -24.0741)
  line L19 (-0.5, -24.0741) -> (-4, -24.0741)
  line L20 (-4, -62.6667) -> (-24.0741, -62.6667)
  line L21 (-24.0741, -62.6667) -> (-24.0741, -61.6667)
  line L22 (-24.0741, -61.6667) -> (-4, -61.6667)
  line L23 (-4, -61.6667) -> (-4, -62.6667)
  line L24 (-4, -62.6667) -> (-5, -62.6667)
  line L25 (-5, -62.6667) -> (-5, -42.5926)
  line L26 (-5, -42.5926) -> (-4, -42.5926)
  line L27 (-4, -42.5926) -> (-4, -62.6667)
  line L28 (-4, -4) -> (-5, -4)
  line L29 (-5, -4) -> (-5, -24.0741)
  line L30 (-5, -24.0741) -> (-4, -24.0741)
  line L31 (-4, -24.0741) -> (-4, -4)
  line L32 (-4, -4) -> (-24.0741, -4)
  line L33 (-24.0741, -4) -> (-24.0741, -5)
  line L34 (-24.0741, -5) -> (-4, -5)
  line L35 (-4, -5) -> (-4, -4)
  line L36 (-62.6667, -4) -> (-61.6667, -4)
  line L37 (-61.6667, -4) -> (-61.6667, -24.0741)
  line L38 (-61.6667, -24.0741) -> (-62.6667, -24.0741)
  line L39 (-62.6667, -24.0741) -> (-62.6667, -4)
  line L40 (-62.6667, -4) -> (-42.5926, -4)
  line L41 (-42.5926, -4) -> (-42.5926, -5)
  line L42 (-42.5926, -5) -> (-62.6667, -5)
  line L43 (-62.6667, -5) -> (-62.6667, -4)
  line L44 (-62.6667, -62.6667) -> (-42.5926, -62.6667)
  line L45 (-42.5926, -62.6667) -> (-42.5926, -61.6667)
  line L46 (-42.5926, -61.6667) -> (-62.6667, -61.6667)
  line L47 (-62.6667, -61.6667) -> (-62.6667, -62.6667)
  line L48 (-62.6667, -62.6667) -> (-61.6667, -62.6667)
  line L49 (-61.6667, -62.6667) -> (-61.6667, -42.5926)
  line L50 (-61.6667, -42.5926) -> (-62.6667, -42.5926)
  line L51 (-62.6667, -42.5926) -> (-62.6667, -62.6667)
  dimension "d495" = 20.0741
  dimension "d496" = 20.0741
  dimension "d497" = 1
  dimension "d498" = 1
  dimension "d499" = 1
  dimension "d500" = 20.0741
  dimension "d501" = 20.0741
  dimension "d502" = 1
  dimension "d503" = 20.0741
  dimension "d504" = 1
  dimension "d505" = 1
  dimension "d506" = 20.0741
  dimension "d507" = 20.0741
  dimension "d508" = 1
  dimension "d509" = 20.0741
  dimension "d510" = 1
  constraint horizontal L20
  constraint vertical L21
  constraint horizontal L22
  constraint vertical L23
  constraint coincident L15.end L16.start
  constraint horizontal L24
  constraint vertical L25
  constraint horizontal L26
  constraint vertical L27
  constraint horizontal L28
  constraint vertical L29
  constraint horizontal L30
  constraint vertical L31
  constraint coincident L0.end L1.start
  constraint horizontal L32
  constraint vertical L33
  constraint horizontal L34
  constraint vertical L35
  constraint horizontal L36
  constraint vertical L37
  constraint horizontal L38
  constraint vertical L39
  constraint coincident L5.end L6.start
  constraint horizontal L40
  constraint vertical L41
  constraint horizontal L42
  constraint vertical L43
  constraint horizontal L44
  constraint vertical L45
  constraint horizontal L46
  constraint vertical L47
  constraint coincident L10.end L11.start
  constraint horizontal L48
  constraint vertical L49
  constraint horizontal L50
  constraint vertical L51
  measures "d495" distance of L10.end L9.end
  measures "d496" distance of L10.end L11.end
  measures "d497" distance of L11.end L45.end
  measures "d498" distance of L49.end L9.end
  measures "d499" distance of L14.end L21.end
  measures "d500" distance of L15.end L14.end
  measures "d501" distance of L15.end L16.end
  measures "d502" distance of L25.end L16.end
  measures "d503" distance of L0.end L1.end
  measures "d504" distance of L1.end L33.end
  measures "d505" distance of L0.end L28.end
  measures "d506" distance of L0.end L0.start
  measures "d507" distance of L5.end L4.end
  measures "d508" distance of L4.end L41.end
  measures "d509" distance of L5.end L6.end
  measures "d510" distance of L37.end L6.end
extrude "Extrude47" cut sketch "Sketch78" against normal blind 4 contours L0 L29 L30 L31 L34 | L0 L1 L28 L29 L31 L32 L34 L35 | L1 L29 L32 L33 L34 | L16 L22 L25 L26 L27 | L15 L16 L20 L22 L23 L24 L25 L27 | L15 L20 L21 L22 L25 | L5 L37 L40 L41 L42 | L5 L6 L36 L37 L39 L40 L42 L43 | L6 L37 L38 L39 L42 | L11 L44 L45 L46 L49 | L10 L11 L44 L46 L47 L48 L49 L51 | L10 L46 L49 L50 L51 bodies 13
sketch "Sketch79" plane through (0, 0, 40) normal (0, 0, 1) x (-1, 0, 0)
  line L0 (-129.3333, -62.6667) -> (-109.2593, -62.6667)
  line L1 (-109.2593, -62.6667) -> (-109.2593, -66.1667)
  line L2 (-109.2593, -66.1667) -> (-90.7407, -66.1667)
  line L3 (-90.7407, -66.1667) -> (-90.7407, -62.6667)
  line L4 (-90.7407, -62.6667) -> (-70.6667, -62.6667)
  line L5 (-70.6667, -62.6667) -> (-70.6667, -42.5926)
  line L6 (-70.6667, -42.5926) -> (-67.1667, -42.5926)
  line L7 (-67.1667, -42.5926) -> (-67.1667, -24.0741)
  line L8 (-67.1667, -24.0741) -> (-70.6667, -24.0741)
  line L9 (-70.6667, -24.0741) -> (-70.6667, -4)
  line L10 (-70.6667, -4) -> (-90.7407, -4)
  line L11 (-90.7407, -4) -> (-90.7407, -0.5)
  line L12 (-90.7407, -0.5) -> (-109.2593, -0.5)
  line L13 (-109.2593, -0.5) -> (-109.2593, -4)
  line L14 (-109.2593, -4) -> (-129.3333, -4)
  line L15 (-129.3333, -4) -> (-129.3333, -24.0741)
  line L16 (-129.3333, -24.0741) -> (-132.8333, -24.0741)
  line L17 (-132.8333, -24.0741) -> (-132.8333, -42.5926)
  line L18 (-132.8333, -42.5926) -> (-129.3333, -42.5926)
  line L19 (-129.3333, -42.5926) -> (-129.3333, -62.6667)
  line L20 (-70.6667, -62.6667) -> (-90.7407, -62.6667)
  line L21 (-90.7407, -62.6667) -> (-90.7407, -61.6667)
  line L22 (-90.7407, -61.6667) -> (-70.6667, -61.6667)
  line L23 (-70.6667, -61.6667) -> (-70.6667, -62.6667)
  line L24 (-70.6667, -62.6667) -> (-71.6667, -62.6667)
  line L25 (-71.6667, -62.6667) -> (-71.6667, -42.5926)
  line L26 (-71.6667, -42.5926) -> (-70.6667, -42.5926)
  line L27 (-70.6667, -42.5926) -> (-70.6667, -62.6667)
  line L28 (-109.2593, -62.6667) -> (-129.3333, -62.6667)
  line L29 (-129.3333, -62.6667) -> (-129.3333, -61.6667)
  line L30 (-129.3333, -61.6667) -> (-109.2593, -61.6667)
  line L31 (-109.2593, -61.6667) -> (-109.2593, -62.6667)
  line L32 (-129.3333, -62.6667) -> (-128.3333, -62.6667)
  line L33 (-128.3333, -62.6667) -> (-128.3333, -42.5926)
  line L34 (-128.3333, -42.5926) -> (-129.3333, -42.5926)
  line L35 (-129.3333, -42.5926) -> (-129.3333, -62.6667)
  line L36 (-129.3333, -4) -> (-128.3333, -4)
  line L37 (-128.3333, -4) -> (-128.3333, -24.0741)
  line L38 (-128.3333, -24.0741) -> (-129.3333, -24.0741)
  line L39 (-129.3333, -24.0741) -> (-129.3333, -4)
  line L40 (-129.3333, -4) -> (-109.2593, -4)
  line L41 (-109.2593, -4) -> (-109.2593, -5)
  line L42 (-109.2593, -5) -> (-129.3333, -5)
  line L43 (-129.3333, -5) -> (-129.3333, -4)
  line L44 (-70.6667, -4) -> (-71.6667, -4)
  line L45 (-71.6667, -4) -> (-71.6667, -24.0741)
  line L46 (-71.6667, -24.0741) -> (-70.6667, -24.0741)
  line L47 (-70.6667, -24.0741) -> (-70.6667, -4)
  line L48 (-70.6667, -4) -> (-90.7407, -4)
  line L49 (-90.7407, -4) -> (-90.7407, -5)
  line L50 (-90.7407, -5) -> (-70.6667, -5)
  line L51 (-70.6667, -5) -> (-70.6667, -4)
  dimension "d513" = 20.0741
  dimension "d514" = 20.0741
  dimension "d515" = 20.0741
  dimension "d516" = 20.0741
  dimension "d517" = 20.0741
  dimension "d518" = 20.0741
  dimension "d519" = 20.0741
  dimension "d520" = 20.0741
  dimension "d521" = 1
  dimension "d522" = 1
  dimension "d523" = 1
  dimension "d524" = 1
  dimension "d525" = 1
  dimension "d526" = 1
  dimension "d527" = 1
  dimension "d528" = 1
  constraint horizontal L20
  constraint vertical L21
  constraint horizontal L22
  constraint vertical L23
  constraint coincident L4.end L5.start
  constraint horizontal L24
  constraint vertical L25
  constraint horizontal L26
  constraint vertical L27
  constraint horizontal L28
  constraint vertical L29
  constraint horizontal L30
  constraint vertical L31
  constraint coincident L0.end L1.start
  constraint horizontal L32
  constraint vertical L33
  constraint horizontal L34
  constraint vertical L35
  constraint coincident L0.start L19.end
  constraint horizontal L36
  constraint vertical L37
  constraint horizontal L38
  constraint vertical L39
  constraint coincident L14.end L15.start
  constraint horizontal L40
  constraint vertical L41
  constraint horizontal L42
  constraint vertical L43
  constraint horizontal L44
  constraint vertical L45
  constraint horizontal L46
  constraint vertical L47
  constraint coincident L9.end L10.start
  constraint horizontal L48
  constraint vertical L49
  constraint horizontal L50
  constraint vertical L51
  measures "d513" distance of L21.end L22.end
  measures "d514" distance of L24.end L25.end
  measures "d515" distance of L29.end L30.end
  measures "d516" distance of L32.end L33.end
  measures "d517" distance of L36.end L37.end
  measures "d518" distance of L41.end L42.end
  measures "d519" distance of L49.end L50.end
  measures "d520" distance of L44.end L45.end
  measures "d521" distance of L25.end L5.end
  measures "d522" distance of L10.end L49.end
  measures "d523" distance of L9.end L44.end
  measures "d524" distance of L36.end L14.end
  measures "d525" distance of L13.end L41.end
  measures "d526" distance of L3.end L21.end
  measures "d527" distance of L0.end L30.end
  measures "d528" distance of L33.end L18.end
extrude "Extrude48" cut sketch "Sketch79" against normal blind 4 contours L0 L19 L28 L29 L30 L32 L33 L35 | L0 L28 L30 L31 L33 | L19 L30 L33 L34 L35 | L4 L20 L21 L22 L25 | L15 L37 L38 L39 L42 | L4 L5 L20 L22 L23 L24 L25 L27 | L14 L15 L36 L37 L39 L40 L42 L43 | L5 L22 L25 L26 L27 | L14 L37 L40 L41 L42 | L9 L45 L46 L47 L50 | L10 L45 L48 L49 L50 | L9 L10 L44 L45 L47 L48 L50 L51 bodies 14
sketch "Sketch80" plane through (0, 0, 40) normal (0, 0, 1) x (-1, 0, 0)
  line L0 (-196, -62.6667) -> (-175.9259, -62.6667)
  line L1 (-175.9259, -62.6667) -> (-175.9259, -66.1667)
  line L2 (-175.9259, -66.1667) -> (-157.4074, -66.1667)
  line L3 (-157.4074, -66.1667) -> (-157.4074, -62.6667)
  line L4 (-157.4074, -62.6667) -> (-137.3333, -62.6667)
  line L5 (-137.3333, -62.6667) -> (-137.3333, -42.5926)
  line L6 (-137.3333, -42.5926) -> (-133.8333, -42.5926)
  line L7 (-133.8333, -42.5926) -> (-133.8333, -24.0741)
  line L8 (-133.8333, -24.0741) -> (-137.3333, -24.0741)
  line L9 (-137.3333, -24.0741) -> (-137.3333, -4)
  line L10 (-137.3333, -4) -> (-157.4074, -4)
  line L11 (-157.4074, -4) -> (-157.4074, -0.5)
  line L12 (-157.4074, -0.5) -> (-175.9259, -0.5)
  line L13 (-175.9259, -0.5) -> (-175.9259, -4)
  line L14 (-175.9259, -4) -> (-196, -4)
  line L15 (-196, -4) -> (-196, -24.0741)
  line L16 (-196, -24.0741) -> (-199.5, -24.0741)
  line L17 (-199.5, -24.0741) -> (-199.5, -42.5926)
  line L18 (-199.5, -42.5926) -> (-196, -42.5926)
  line L19 (-196, -42.5926) -> (-196, -62.6667)
  line L20 (-137.3333, -62.6667) -> (-157.4074, -62.6667)
  line L21 (-157.4074, -62.6667) -> (-157.4074, -61.6667)
  line L22 (-157.4074, -61.6667) -> (-137.3333, -61.6667)
  line L23 (-137.3333, -61.6667) -> (-137.3333, -62.6667)
  line L24 (-137.3333, -62.6667) -> (-138.3333, -62.6667)
  line L25 (-138.3333, -62.6667) -> (-138.3333, -42.5926)
  line L26 (-138.3333, -42.5926) -> (-137.3333, -42.5926)
  line L27 (-137.3333, -42.5926) -> (-137.3333, -62.6667)
  line L28 (-137.3333, -4) -> (-138.3333, -4)
  line L29 (-138.3333, -4) -> (-138.3333, -24.0741)
  line L30 (-138.3333, -24.0741) -> (-137.3333, -24.0741)
  line L31 (-137.3333, -24.0741) -> (-137.3333, -4)
  line L32 (-137.3333, -4) -> (-157.4074, -4)
  line L33 (-157.4074, -4) -> (-157.4074, -5)
  line L34 (-157.4074, -5) -> (-137.3333, -5)
  line L35 (-137.3333, -5) -> (-137.3333, -4)
  line L36 (-196, -4) -> (-195, -4)
  line L37 (-195, -4) -> (-195, -24.0741)
  line L38 (-195, -24.0741) -> (-196, -24.0741)
  line L39 (-196, -24.0741) -> (-196, -4)
  line L40 (-196, -4) -> (-175.9259, -4)
  line L41 (-175.9259, -4) -> (-175.9259, -5)
  line L42 (-175.9259, -5) -> (-196, -5)
  line L43 (-196, -5) -> (-196, -4)
  line L44 (-175.9259, -62.6667) -> (-196, -62.6667)
  line L45 (-196, -62.6667) -> (-196, -61.6667)
  line L46 (-196, -61.6667) -> (-175.9259, -61.6667)
  line L47 (-175.9259, -61.6667) -> (-175.9259, -62.6667)
  line L48 (-196, -62.6667) -> (-195, -62.6667)
  line L49 (-195, -62.6667) -> (-195, -42.5926)
  line L50 (-195, -42.5926) -> (-196, -42.5926)
  line L51 (-196, -42.5926) -> (-196, -62.6667)
  dimension "d531" = 1
  dimension "d532" = 1
  dimension "d533" = 1
  dimension "d534" = 1
  dimension "d535" = 1
  dimension "d536" = 1
  dimension "d537" = 1
  dimension "d538" = 1
  dimension "d539" = 20.0741
  dimension "d540" = 20.0741
  dimension "d541" = 20.0741
  dimension "d542" = 20.0741
  dimension "d543" = 20.0741
  dimension "d544" = 20.0741
  dimension "d545" = 20.0741
  dimension "d546" = 20.0741
  constraint horizontal L20
  constraint vertical L21
  constraint horizontal L22
  constraint vertical L23
  constraint coincident L4.end L5.start
  constraint horizontal L24
  constraint vertical L25
  constraint horizontal L26
  constraint vertical L27
  constraint horizontal L28
  constraint vertical L29
  constraint horizontal L30
  constraint vertical L31
  constraint coincident L9.end L10.start
  constraint horizontal L32
  constraint vertical L33
  constraint horizontal L34
  constraint vertical L35
  constraint horizontal L36
  constraint vertical L37
  constraint horizontal L38
  constraint vertical L39
  constraint coincident L14.end L15.start
  constraint horizontal L40
  constraint vertical L41
  constraint horizontal L42
  constraint vertical L43
  constraint horizontal L44
  constraint vertical L45
  constraint horizontal L46
  constraint vertical L47
  constraint coincident L0.end L1.start
  constraint horizontal L48
  constraint vertical L49
  constraint horizontal L50
  constraint vertical L51
  constraint coincident L0.start L19.end
  measures "d531" distance of L3.end L21.end
  measures "d532" distance of L0.end L46.end
  measures "d533" distance of L49.end L18.end
  measures "d534" distance of L37.end L15.end
  measures "d535" distance of L13.end L41.end
  measures "d536" distance of L10.end L33.end
  measures "d537" distance of L29.end L8.end
  measures "d538" distance of L25.end L5.end
  measures "d539" distance of L21.end L22.end
  measures "d540" distance of L45.end L46.end
  measures "d541" distance of L41.end L42.end
  measures "d542" distance of L33.end L34.end
  measures "d543" distance of L24.end L25.end
  measures "d544" distance of L48.end L49.end
  measures "d545" distance of L14.end L15.end
  measures "d546" distance of L9.end L8.end
extrude "Extrude49" cut sketch "Sketch80" against normal blind 4 contours L0 L19 L44 L45 L46 L48 L49 L51 | L0 L44 L46 L47 L49 | L19 L46 L49 L50 L51 | L4 L20 L21 L22 L25 | L15 L37 L38 L39 L42 | L4 L5 L20 L22 L23 L24 L25 L27 | L14 L15 L36 L37 L39 L40 L42 L43 | L5 L22 L25 L26 L27 | L14 L37 L40 L41 L42 | L9 L29 L30 L31 L34 | L10 L29 L32 L33 L34 | L9 L10 L28 L29 L31 L32 L34 L35 bodies 15